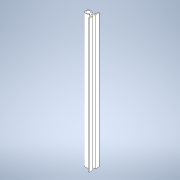
# Autodesk Inventor part: linear_drive_new
Saved by Autodesk Inventor 2022 (Build 260153000, 153)
## iProperties
Created: 2022-08-12
Part Number: linear_drive_new
Material: Generic
Document SubType Name: Modeling
Designer: Alok
Density: 1 g/cm^3
Appearance: Default
Author: Alok
Autodesk Inventor part; units mm, degrees
ref_plane "YZ Plane" through (0, 0, 0) normal (1, 0, 0) x (0, 1, 0)
ref_plane "XZ Plane" through (0, 0, 0) normal (0, 1, 0) x (-1, 0, 0)
ref_plane "XY Plane" through (0, 0, 0) normal (0, 0, 1) x (1, 0, 0)
sketch "Sketch1" plane through (0, 0, 0) normal (0, 1, 0) x (-1, 0, 0)
  line L0 (0, 0) -> (0, -37.5)
  line L1 (0, 0) -> (0, 37.5)
  line L2 (0, 37.5) -> (7, 37.5)
  line L3 (7, 37.5) -> (7, 17.5)
  line L4 (0, -37.5) -> (7, -37.5)
  line L5 (7, -37.5) -> (7, -17.5)
  line L6 (7, 0) -> (27, 0) construction
  line L7 (27, -10) -> (7, -17.5)
  line L8 (7, 17.5) -> (27, 10)
  line L9 (27, 0) -> (47, 0)
  circle A0 centre (47, 0) radius 20
  circle A1 centre (47, 0) radius 13.5
  line L10 (27, 10) -> (29.224, 9.166)
  line L11 (27, -10) -> (29.224, -9.166)
  line L12 (0, 17.5) -> (0, 10.5)
  line L13 (20, 0) -> (20, 4)
  line L14 (0, 10.5) -> (20, 4)
  line L15 (0, -17.5) -> (0, -10.5)
  line L16 (20, 0) -> (20, -4)
  line L17 (20, -4) -> (0, -10.5)
  dimension "d0" = 37.5
  dimension "d1" = 37.5
  dimension "d2" = 7
  dimension "d3" = 20
  dimension "d4" = 20
  dimension "d11" = 27
  dimension "d12" = 7
  dimension "d14" = 4
  dimension "d16" = 7
  dimension "d18" = 4
  constraints: 36 end point, 6 point on line, 4 horizontal, 3 perpendicular, 3 vertical, 2 centre point, 2 coincident, 2 point on circle
  measures "d0" distance of L0.start L1.end
  measures "d1" distance of L0.start L0.end
  measures "d2" distance of L1.end L2.end
  measures "d3" distance of L2.end L3.end
  measures "d4" distance of L4.end L5.end
  measures "d11" diameter of A1
  measures "d12" distance of L12.start L12.end
  measures "d14" distance of L13.start L13.end
  measures "d16" distance of L15.start L15.end
  measures "d18" distance of L13.start L16.end
extrude "Extrusion1" add sketch "Sketch1" along normal blind 1030 contours L17 L16 L13 L14 L1 L2 L3 L8 L10 A0 L11 L7 L5 L4 L0 | A0
sketch "Sketch2" plane through (0, 1030, 0) normal (0, 1, 0) x (1, 0, 0)
  point P0 (0, 0)
body "Solid1"
